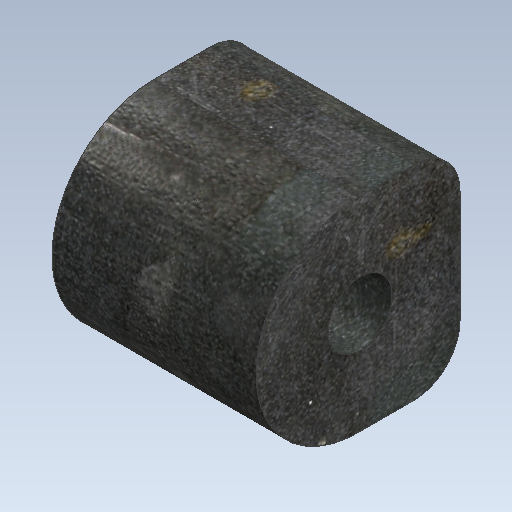
# Autodesk Inventor part: jakis_modulxD
Saved by Autodesk Inventor 2021 (Build 250183000, 183)
## iProperties
Created: 2021-06-18
Part Number: jakis_modulxD
Material: Stal
Document SubType Name: Modeling
Designer: Wojciech Wołczek
Density: 7.85 g/cm^3
Appearance: Płyta
Author: Wojciech Wołczek
Autodesk Inventor part; units mm, degrees
ref_plane "YZ Plane" through (0, 0, 0) normal (1, 0, 0) x (0, 1, 0)
ref_plane "XZ Plane" through (0, 0, 0) normal (0, 1, 0) x (-1, 0, 0)
ref_plane "XY Plane" through (0, 0, 0) normal (0, 0, 1) x (1, 0, 0)
sketch "Szkic3" plane through (0, 0, 0) normal (0, 0, 1) x (1, 0, 0)
  line L0 (-40, -40) -> (40, -40)
  line L1 (40, -40) -> (40, 40)
  line L2 (40, 40) -> (-40, 40)
  line L3 (-40, 40) -> (-40, -40)
  line L4 (-40, -40) -> (40, 40) construction
  line L5 (40, -40) -> (-40, 40) construction
  point P0 (0, 0)
  dimension "d8" = 80
  dimension "d9" = 80
  constraints: 12 end point, 2 midpoint, 2 parallel, 1 horizontal, 1 perpendicular
  measures "d8" distance of L2.end L1.end
  measures "d9" distance of L1.end L0.end
extrude "Wyciągnięcie proste3" add sketch "Szkic3" along normal blind 80
fillet "Zaokrąglenie2" radius 18 2 edges at (0, 40, 0) (0, -40, 0)
fillet "Zaokrąglenie3" radius 40 2 edges at (0, 40, 80) (0, -40, 80)
sketch "Szkic4" plane through (40, -22, 0) normal (1, 0, 0) x (0, 0, -1)
  circle A0 centre (-39.1753, 22) radius 12.5
  point P0 (0, 22)
  dimension "d14" = 25
  constraints: 1 centre point
  measures "d14" diameter of A0
extrude "Wyciągnięcie proste4" cut sketch "Szkic4" against normal through all
